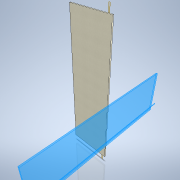
# Autodesk Inventor part: sciana
Saved by Autodesk Inventor 2021 (Build 250183000, 183)
## iProperties
Created: 2021-04-01
Part Number: sciana
Material: MDF — płyta pilśniowa o średniej gęstości
Document SubType Name: Modeling
Designer: Wojciech Wołczek
Density: 0.8 g/cm^3
Appearance: Tektura — falista
Mass: 17280 g
Surface Area: 24936 cm^2
Volume: 21600 cm^3
Author: Wojciech Wołczek
Autodesk Inventor part; units mm, degrees
ref_plane "YZ Plane" through (0, 0, 0) normal (1, 0, 0) x (0, 1, 0)
ref_plane "XZ Plane" through (0, 0, 0) normal (0, 1, 0) x (-1, 0, 0)
ref_plane "XY Plane" through (0, 0, 0) normal (0, 0, 1) x (1, 0, 0)
ref_plane "Płaszczyzna konstrukcyjna1" through (0, 0, 0) normal (0, 0, 1) x (1, 0, 0)
sketch "Szkic1" plane through (0, 0, 0) normal (0, 0, 1) x (1, 0, 0)
  line L0 (50, 0) -> (-550, 0)
  line L1 (-550, 0) -> (-550, 2000)
  line L2 (-550, 2000) -> (50, 2000)
  line L3 (50, 2000) -> (50, 0)
  line L4 (0, 0) -> (0, 2000) projected
  dimension "d0" = 600
  dimension "d1" = 2000
  dimension "d2" = 50
  constraints: 8 end point, 2 parallel, 1 horizontal, 1 perpendicular
  measures "d0" distance of L1.end L2.end
  measures "d1" distance of L0.end L1.end
  measures "d2" distance between parallel lines of L3 L4
extrude "Wyciągnięcie proste1" add sketch "Szkic1" along normal blind 18
